Autodesk Inventor part; units mm, degrees
(part 2 of 2)
sketch "スケッチ3" plane through (0, 0, 4) normal (0, 0, 1) x (1, 0, 0)
  circle A0 centre (148.5, 105.0001) radius 6.8 projected
  arc A1 (157.8649, 90.2168) -> (159.6658, 91.5252) centre (148.5, 105.0001) ccw projected
  line L0 (159.6658, 91.5252) -> (160.4913, 90.529) projected
  arc A2 (160.4913, 90.529) -> (160.7031, 90.3266) centre (161.9356, 91.8285) ccw projected
  arc A3 (160.7031, 90.3266) -> (161.5747, 89.744) centre (164.1012, 94.4672) ccw projected
  arc A4 (161.5747, 89.744) -> (163.5573, 88.9603) centre (165.9672, 97.9557) ccw projected
  arc A5 (163.5573, 88.9603) -> (164.5398, 89.9428) centre (148.5, 105.0001) ccw projected
  arc A6 (164.5398, 89.9428) -> (163.7561, 91.9254) centre (155.5444, 87.5329) ccw projected
  arc A7 (163.7561, 91.9254) -> (163.1735, 92.797) centre (159.0329, 89.3989) ccw projected
  arc A8 (163.1735, 92.797) -> (162.9711, 93.0088) centre (161.6716, 91.5644) ccw projected
  line L1 (162.9711, 93.0088) -> (161.9749, 93.8343) projected
  arc A9 (161.9749, 93.8343) -> (163.2833, 95.6351) centre (148.5, 105.0001) ccw projected
  line L2 (163.2833, 95.6351) -> (164.3763, 94.9428) projected
  arc A10 (164.3763, 94.9428) -> (164.6402, 94.8158) centre (165.3483, 96.625) ccw projected
  arc A11 (164.6402, 94.8158) -> (165.6492, 94.531) centre (166.5924, 99.8038) ccw projected
  arc A12 (165.6492, 94.531) -> (167.7769, 94.3983) centre (167.2891, 103.6981) ccw projected
  arc A13 (167.7769, 94.3983) -> (168.4077, 95.6364) centre (148.5, 105.0001) ccw projected
  arc A14 (168.4077, 95.6364) -> (167.0497, 97.2797) centre (160.5973, 90.5647) ccw projected
  arc A15 (167.0497, 97.2797) -> (166.2263, 97.9286) centre (163.3384, 93.4173) ccw projected
  arc A16 (166.2263, 97.9286) -> (165.9684, 98.0675) centre (165.1788, 96.2923) ccw projected
  line L3 (165.9684, 98.0675) -> (164.7658, 98.5448) projected
  arc A17 (164.7658, 98.5448) -> (165.4537, 100.6618) centre (148.5, 105.0001) ccw projected
  line L4 (165.4537, 100.6618) -> (166.7071, 100.341) projected
  arc A18 (166.7071, 100.341) -> (166.9974, 100.3018) centre (167.1118, 102.2413) ccw projected
  arc A19 (166.9974, 100.3018) -> (168.045, 100.3428) centre (167.3127, 105.649) ccw projected
  arc A20 (168.045, 100.3428) -> (170.1096, 100.8741) centre (166.7718, 109.568) ccw projected
  arc A21 (170.1096, 100.8741) -> (170.327, 102.2465) centre (148.5, 105.0001) ccw projected
  arc A22 (170.327, 102.2465) -> (168.5276, 103.3897) centre (164.466, 95.0095) ccw projected
  arc A23 (168.5276, 103.3897) -> (167.5439, 103.7525) centre (166.1914, 98.5696) ccw projected
  arc A24 (167.5439, 103.7525) -> (167.2557, 103.8049) centre (167.0533, 101.8725) ccw projected
  line L5 (167.2557, 103.8049) -> (165.9645, 103.8871) projected
  arc A25 (165.9645, 103.8871) -> (165.9645, 106.1131) centre (148.5, 105.0001) ccw projected
  line L6 (165.9645, 106.1131) -> (167.2557, 106.1954) projected
  arc A26 (167.2557, 106.1954) -> (167.5439, 106.2478) centre (167.0533, 108.1277) ccw projected
  arc A27 (167.5439, 106.2478) -> (168.5276, 106.6105) centre (166.1914, 111.4307) ccw projected
  arc A28 (168.5276, 106.6105) -> (170.327, 107.7538) centre (164.466, 114.9908) ccw projected
  arc A29 (170.327, 107.7538) -> (170.1096, 109.1262) centre (148.5, 105.0001) ccw projected
  arc A30 (170.1096, 109.1262) -> (168.045, 109.6574) centre (166.7718, 100.4322) ccw projected
  arc A31 (168.045, 109.6574) -> (166.9974, 109.6984) centre (167.3127, 104.3513) ccw projected
  arc A32 (166.9974, 109.6984) -> (166.7071, 109.6592) centre (167.1118, 107.7589) ccw projected
  line L7 (166.7071, 109.6592) -> (165.4537, 109.3385) projected
  arc A33 (165.4537, 109.3385) -> (164.7658, 111.4555) centre (148.5, 105.0001) ccw projected
  line L8 (164.7658, 111.4555) -> (165.9684, 111.9328) projected
  arc A34 (165.9684, 111.9328) -> (166.2263, 112.0716) centre (165.1788, 113.708) ccw projected
  arc A35 (166.2263, 112.0716) -> (167.0497, 112.7206) centre (163.3384, 116.5829) ccw projected
  arc A36 (167.0497, 112.7206) -> (168.4077, 114.3639) centre (160.5973, 119.4356) ccw projected
  arc A37 (168.4077, 114.3639) -> (167.7769, 115.602) centre (148.5, 105.0001) ccw projected
  arc A38 (167.7769, 115.602) -> (165.6492, 115.4692) centre (167.2891, 106.3021) ccw projected
  arc A39 (165.6492, 115.4692) -> (164.6402, 115.1845) centre (166.5924, 110.1965) ccw projected
  arc A40 (164.6402, 115.1845) -> (164.3763, 115.0575) centre (165.3483, 113.3753) ccw projected
  line L9 (164.3763, 115.0575) -> (163.2833, 114.3651) projected
  arc A41 (163.2833, 114.3651) -> (161.9749, 116.166) centre (148.5, 105.0001) ccw projected
  line L10 (161.9749, 116.166) -> (162.9711, 116.9915) projected
  arc A42 (162.9711, 116.9915) -> (163.1735, 117.2033) centre (161.6716, 118.4358) ccw projected
  arc A43 (163.1735, 117.2033) -> (163.7561, 118.0749) centre (159.0329, 120.6013) ccw projected
  arc A44 (163.7561, 118.0749) -> (164.5398, 120.0574) centre (155.5444, 122.4673) ccw projected
  arc A45 (164.5398, 120.0574) -> (163.5573, 121.04) centre (148.5, 105.0001) ccw projected
  arc A46 (163.5573, 121.04) -> (161.5747, 120.2563) centre (165.9672, 112.0445) ccw projected
  arc A47 (161.5747, 120.2563) -> (160.7031, 119.6736) centre (164.1012, 115.533) ccw projected
  arc A48 (160.7031, 119.6736) -> (160.4913, 119.4713) centre (161.9356, 118.1718) ccw projected
  line L11 (160.4913, 119.4713) -> (159.6658, 118.4751) projected
  arc A49 (159.6658, 118.4751) -> (157.8649, 119.7835) centre (148.5, 105.0001) ccw projected
  line L12 (157.8649, 119.7835) -> (158.5573, 120.8764) projected
  arc A50 (158.5573, 120.8764) -> (158.6843, 121.1404) centre (156.8751, 121.8485) ccw projected
  arc A51 (158.6843, 121.1404) -> (158.9691, 122.1494) centre (153.6963, 123.0926) ccw projected
  arc A52 (158.9691, 122.1494) -> (159.1018, 124.2771) centre (149.8019, 123.7893) ccw projected
  arc A53 (159.1018, 124.2771) -> (157.8637, 124.9079) centre (148.5, 105.0001) ccw projected
  arc A54 (157.8637, 124.9079) -> (156.2204, 123.5499) centre (162.9354, 117.0974) ccw projected
  arc A55 (156.2204, 123.5499) -> (155.5715, 122.7265) centre (160.0827, 119.8386) ccw projected
  arc A56 (155.5715, 122.7265) -> (155.4326, 122.4686) centre (157.2078, 121.679) ccw projected
  line L13 (155.4326, 122.4686) -> (154.9553, 121.266) projected
  arc A57 (154.9553, 121.266) -> (152.8383, 121.9539) centre (148.5, 105.0001) ccw projected
  line L14 (152.8383, 121.9539) -> (153.159, 123.2073) projected
  arc A58 (153.159, 123.2073) -> (153.1983, 123.4975) centre (151.2588, 123.6119) ccw projected
  arc A59 (153.1983, 123.4975) -> (153.1573, 124.5452) centre (147.8511, 123.8129) ccw projected
  arc A60 (153.1573, 124.5452) -> (152.626, 126.6097) centre (143.9321, 123.272) ccw projected
  arc A61 (152.626, 126.6097) -> (151.2536, 126.8271) centre (148.5, 105.0001) ccw projected
  arc A62 (151.2536, 126.8271) -> (150.1104, 125.0278) centre (158.4906, 120.9661) ccw projected
  arc A63 (150.1104, 125.0278) -> (149.7476, 124.0441) centre (154.9305, 122.6916) ccw projected
  arc A64 (149.7476, 124.0441) -> (149.6952, 123.7559) centre (151.6276, 123.5535) ccw projected
  line L15 (149.6952, 123.7559) -> (149.613, 122.4647) projected
  arc A65 (149.613, 122.4647) -> (147.387, 122.4647) centre (148.5, 105.0001) ccw projected
  line L16 (147.387, 122.4647) -> (147.3047, 123.7559) projected
  arc A66 (147.3047, 123.7559) -> (147.2523, 124.0441) centre (145.3724, 123.5535) ccw projected
  arc A67 (147.2523, 124.0441) -> (146.8896, 125.0278) centre (142.0694, 122.6916) ccw projected
  arc A68 (146.8896, 125.0278) -> (145.7463, 126.8271) centre (138.5093, 120.9661) ccw projected
  arc A69 (145.7463, 126.8271) -> (144.3739, 126.6097) centre (148.5, 105.0001) ccw projected
  arc A70 (144.3739, 126.6097) -> (143.8427, 124.5452) centre (153.0679, 123.272) ccw projected
  arc A71 (143.8427, 124.5452) -> (143.8017, 123.4975) centre (149.1488, 123.8129) ccw projected
  arc A72 (143.8017, 123.4975) -> (143.8409, 123.2073) centre (145.7412, 123.6119) ccw projected
  line L17 (143.8409, 123.2073) -> (144.1616, 121.9539) projected
  arc A73 (144.1616, 121.9539) -> (142.0446, 121.266) centre (148.5, 105.0001) ccw projected
  line L18 (142.0446, 121.266) -> (141.5673, 122.4686) projected
  arc A74 (141.5673, 122.4686) -> (141.4285, 122.7265) centre (139.7921, 121.679) ccw projected
  arc A75 (141.4285, 122.7265) -> (140.7795, 123.5499) centre (136.9172, 119.8386) ccw projected
  arc A76 (140.7795, 123.5499) -> (139.1362, 124.9079) centre (134.0645, 117.0974) ccw projected
  arc A77 (139.1362, 124.9079) -> (137.8981, 124.2771) centre (148.5, 105.0001) ccw projected
  arc A78 (137.8981, 124.2771) -> (138.0309, 122.1494) centre (147.198, 123.7893) ccw projected
  arc A79 (138.0309, 122.1494) -> (138.3156, 121.1404) centre (143.3036, 123.0926) ccw projected
  arc A80 (138.3156, 121.1404) -> (138.4426, 120.8764) centre (140.1248, 121.8485) ccw projected
  line L19 (138.4426, 120.8764) -> (139.135, 119.7835) projected
  arc A81 (139.135, 119.7835) -> (137.3341, 118.4751) centre (148.5, 105.0001) ccw projected
  line L20 (137.3341, 118.4751) -> (136.5086, 119.4713) projected
  arc A82 (136.5086, 119.4713) -> (136.2968, 119.6736) centre (135.0643, 118.1718) ccw projected
  arc A83 (136.2968, 119.6736) -> (135.4252, 120.2563) centre (132.8988, 115.533) ccw projected
  arc A84 (135.4252, 120.2563) -> (133.4426, 121.04) centre (131.0328, 112.0445) ccw projected
  arc A85 (133.4426, 121.04) -> (132.4601, 120.0574) centre (148.5, 105.0001) ccw projected
  arc A86 (132.4601, 120.0574) -> (133.2438, 118.0749) centre (141.4555, 122.4673) ccw projected
  arc A87 (133.2438, 118.0749) -> (133.8264, 117.2033) centre (137.967, 120.6013) ccw projected
  arc A88 (133.8264, 117.2033) -> (134.0288, 116.9915) centre (135.3283, 118.4358) ccw projected
  line L21 (134.0288, 116.9915) -> (135.025, 116.166) projected
  arc A89 (135.025, 116.166) -> (133.7166, 114.3651) centre (148.5, 105.0001) ccw projected
  line L22 (133.7166, 114.3651) -> (132.6237, 115.0575) projected
  arc A90 (132.6237, 115.0575) -> (132.3597, 115.1845) centre (131.6516, 113.3753) ccw projected
  arc A91 (132.3597, 115.1845) -> (131.3507, 115.4692) centre (130.4075, 110.1965) ccw projected
  arc A92 (131.3507, 115.4692) -> (129.223, 115.602) centre (129.7108, 106.3021) ccw projected
  arc A93 (129.223, 115.602) -> (128.5922, 114.3639) centre (148.5, 105.0001) ccw projected
  arc A94 (128.5922, 114.3639) -> (129.9502, 112.7206) centre (136.4027, 119.4356) ccw projected
  arc A95 (129.9502, 112.7206) -> (130.7736, 112.0716) centre (133.6615, 116.5829) ccw projected
  arc A96 (130.7736, 112.0716) -> (131.0315, 111.9328) centre (131.8211, 113.708) ccw projected
  line L23 (131.0315, 111.9328) -> (132.2341, 111.4555) projected
  arc A97 (132.2341, 111.4555) -> (131.5462, 109.3385) centre (148.5, 105.0001) ccw projected
  line L24 (131.5462, 109.3385) -> (130.2928, 109.6592) projected
  arc A98 (130.2928, 109.6592) -> (130.0025, 109.6984) centre (129.8882, 107.7589) ccw projected
  arc A99 (130.0025, 109.6984) -> (128.9549, 109.6574) centre (129.6872, 104.3513) ccw projected
  arc A100 (128.9549, 109.6574) -> (126.8903, 109.1262) centre (130.2281, 100.4322) ccw projected
  arc A101 (126.8903, 109.1262) -> (126.673, 107.7538) centre (148.5, 105.0001) ccw projected
  arc A102 (126.673, 107.7538) -> (128.4723, 106.6105) centre (132.5339, 114.9908) ccw projected
  arc A103 (128.4723, 106.6105) -> (129.456, 106.2478) centre (130.8085, 111.4307) ccw projected
  arc A104 (129.456, 106.2478) -> (129.7442, 106.1954) centre (129.9466, 108.1277) ccw projected
  line L25 (129.7442, 106.1954) -> (131.0354, 106.1131) projected
  arc A105 (131.0354, 106.1131) -> (131.0354, 103.8871) centre (148.5, 105.0001) ccw projected
  line L26 (131.0354, 103.8871) -> (129.7442, 103.8049) projected
  arc A106 (129.7442, 103.8049) -> (129.456, 103.7525) centre (129.9466, 101.8725) ccw projected
  arc A107 (129.456, 103.7525) -> (128.4723, 103.3897) centre (130.8085, 98.5696) ccw projected
  arc A108 (128.4723, 103.3897) -> (126.673, 102.2465) centre (132.5339, 95.0095) ccw projected
  arc A109 (126.673, 102.2465) -> (126.8903, 100.8741) centre (148.5, 105.0001) ccw projected
  arc A110 (126.8903, 100.8741) -> (128.9549, 100.3428) centre (130.2281, 109.568) ccw projected
  arc A111 (128.9549, 100.3428) -> (130.0025, 100.3018) centre (129.6872, 105.649) ccw projected
  arc A112 (130.0025, 100.3018) -> (130.2928, 100.341) centre (129.8882, 102.2413) ccw projected
  line L27 (130.2928, 100.341) -> (131.5462, 100.6618) projected
  arc A113 (131.5462, 100.6618) -> (132.2341, 98.5448) centre (148.5, 105.0001) ccw projected
  line L28 (132.2341, 98.5448) -> (131.0315, 98.0675) projected
  arc A114 (131.0315, 98.0675) -> (130.7736, 97.9286) centre (131.8211, 96.2923) ccw projected
  arc A115 (130.7736, 97.9286) -> (129.9502, 97.2797) centre (133.6615, 93.4173) ccw projected
  arc A116 (129.9502, 97.2797) -> (128.5922, 95.6364) centre (136.4027, 90.5647) ccw projected
  arc A117 (128.5922, 95.6364) -> (129.223, 94.3983) centre (148.5, 105.0001) ccw projected
  arc A118 (129.223, 94.3983) -> (131.3507, 94.531) centre (129.7108, 103.6981) ccw projected
  arc A119 (131.3507, 94.531) -> (132.3597, 94.8158) centre (130.4075, 99.8038) ccw projected
  arc A120 (132.3597, 94.8158) -> (132.6237, 94.9428) centre (131.6516, 96.625) ccw projected
  line L29 (132.6237, 94.9428) -> (133.7166, 95.6351) projected
  arc A121 (133.7166, 95.6351) -> (135.025, 93.8343) centre (148.5, 105.0001) ccw projected
  line L30 (135.025, 93.8343) -> (134.0288, 93.0088) projected
  arc A122 (134.0288, 93.0088) -> (133.8264, 92.797) centre (135.3283, 91.5644) ccw projected
  arc A123 (133.8264, 92.797) -> (133.2438, 91.9254) centre (137.967, 89.3989) ccw projected
  arc A124 (133.2438, 91.9254) -> (132.4601, 89.9428) centre (141.4555, 87.5329) ccw projected
  arc A125 (132.4601, 89.9428) -> (133.4426, 88.9603) centre (148.5, 105.0001) ccw projected
  arc A126 (133.4426, 88.9603) -> (135.4252, 89.744) centre (131.0328, 97.9557) ccw projected
  arc A127 (135.4252, 89.744) -> (136.2968, 90.3266) centre (132.8988, 94.4672) ccw projected
  arc A128 (136.2968, 90.3266) -> (136.5086, 90.529) centre (135.0643, 91.8285) ccw projected
  line L31 (136.5086, 90.529) -> (137.3341, 91.5252) projected
  arc A129 (137.3341, 91.5252) -> (139.135, 90.2168) centre (148.5, 105.0001) ccw projected
  line L32 (139.135, 90.2168) -> (138.4426, 89.1238) projected
  arc A130 (138.4426, 89.1238) -> (138.3156, 88.8599) centre (140.1248, 88.1518) ccw projected
  arc A131 (138.3156, 88.8599) -> (138.0309, 87.8509) centre (143.3036, 86.9076) ccw projected
  arc A132 (138.0309, 87.8509) -> (137.8981, 85.7232) centre (147.198, 86.211) ccw projected
  arc A133 (137.8981, 85.7232) -> (139.1362, 85.0923) centre (148.5, 105.0001) ccw projected
  arc A134 (139.1362, 85.0923) -> (140.7795, 86.4504) centre (134.0645, 92.9028) ccw projected
  arc A135 (140.7795, 86.4504) -> (141.4285, 87.2738) centre (136.9172, 90.1617) ccw projected
  arc A136 (141.4285, 87.2738) -> (141.5673, 87.5317) centre (139.7921, 88.3213) ccw projected
  line L33 (141.5673, 87.5317) -> (142.0446, 88.7343) projected
  arc A137 (142.0446, 88.7343) -> (144.1616, 88.0464) centre (148.5, 105.0001) ccw projected
  line L34 (144.1616, 88.0464) -> (143.8409, 86.793) projected
  arc A138 (143.8409, 86.793) -> (143.8017, 86.5027) centre (145.7412, 86.3883) ccw projected
  arc A139 (143.8017, 86.5027) -> (143.8427, 85.4551) centre (149.1488, 86.1874) ccw projected
  arc A140 (143.8427, 85.4551) -> (144.3739, 83.3905) centre (153.0679, 86.7283) ccw projected
  arc A141 (144.3739, 83.3905) -> (145.7463, 83.1731) centre (148.5, 105.0001) ccw projected
  arc A142 (145.7463, 83.1731) -> (146.8896, 84.9725) centre (138.5093, 89.0341) ccw projected
  arc A143 (146.8896, 84.9725) -> (147.2523, 85.9562) centre (142.0694, 87.3087) ccw projected
  arc A144 (147.2523, 85.9562) -> (147.3047, 86.2444) centre (145.3724, 86.4467) ccw projected
  line L35 (147.3047, 86.2444) -> (147.387, 87.5356) projected
  arc A145 (147.387, 87.5356) -> (149.613, 87.5356) centre (148.5, 105.0001) ccw projected
  line L36 (149.613, 87.5356) -> (149.6952, 86.2444) projected
  arc A146 (149.6952, 86.2444) -> (149.7476, 85.9562) centre (151.6276, 86.4467) ccw projected
  arc A147 (149.7476, 85.9562) -> (150.1104, 84.9725) centre (154.9305, 87.3087) ccw projected
  arc A148 (150.1104, 84.9725) -> (151.2536, 83.1731) centre (158.4906, 89.0341) ccw projected
  arc A149 (151.2536, 83.1731) -> (152.626, 83.3905) centre (148.5, 105.0001) ccw projected
  arc A150 (152.626, 83.3905) -> (153.1573, 85.4551) centre (143.9321, 86.7283) ccw projected
  arc A151 (153.1573, 85.4551) -> (153.1983, 86.5027) centre (147.8511, 86.1874) ccw projected
  arc A152 (153.1983, 86.5027) -> (153.159, 86.793) centre (151.2588, 86.3883) ccw projected
  line L37 (153.159, 86.793) -> (152.8383, 88.0464) projected
  arc A153 (152.8383, 88.0464) -> (154.9553, 88.7343) centre (148.5, 105.0001) ccw projected
  line L38 (154.9553, 88.7343) -> (155.4326, 87.5317) projected
  arc A154 (155.4326, 87.5317) -> (155.5715, 87.2738) centre (157.2078, 88.3213) ccw projected
  arc A155 (155.5715, 87.2738) -> (156.2204, 86.4504) centre (160.0827, 90.1617) ccw projected
  arc A156 (156.2204, 86.4504) -> (157.8637, 85.0923) centre (162.9354, 92.9028) ccw projected
  arc A157 (157.8637, 85.0923) -> (159.1018, 85.7232) centre (148.5, 105.0001) ccw projected
  arc A158 (159.1018, 85.7232) -> (158.9691, 87.8509) centre (149.8019, 86.211) ccw projected
  arc A159 (158.9691, 87.8509) -> (158.6843, 88.8599) centre (153.6963, 86.9076) ccw projected
  arc A160 (158.6843, 88.8599) -> (158.5573, 89.1238) centre (156.8751, 88.1518) ccw projected
  line L39 (158.5573, 89.1238) -> (157.8649, 90.2168) projected
  circle A161 centre (148.5, 105.0001) radius 13.5
  circle A162 centre (148.5, 105.0001) radius 10
  circle A163 centre (148.5, 105.0001) radius 6 projected
  line L40 (147, 119.6736) -> (147, 90.1617)
  line L41 (150, 119.9822) -> (150, 90.1617)
  line L42 (132.8988, 106.5001) -> (164.1012, 106.5001)
  line L43 (133.4426, 103.5001) -> (164.5398, 103.5001)
  point P0 (0, 0)
  point P1 (138.6131, 103.5001)
  point P2 (135.0836, 103.5001)
  point P3 (147, 91.5837)
  point P4 (147, 95.1133)
  point P5 (161.9164, 103.5001)
  point P6 (158.3868, 103.5001)
  point P7 (150, 95.1133)
  point P8 (150, 91.5837)
  point P9 (158.3868, 106.5001)
  point P10 (161.9164, 106.5001)
  point P11 (150, 118.4165)
  point P12 (150, 114.887)
  point P13 (135.0836, 106.5001)
  point P14 (138.6131, 106.5001)
  point P15 (147, 114.887)
  point P16 (147, 118.4165)
  dimension "d8" = 4
  dimension "d9" = 4
  dimension "d10" = 1.5
  dimension "d11" = 3
  dimension "d12" = 1.5
  dimension "d13" = 3
  constraints: 8 end point, 2 centre point, 2 coincident, 2 vertical, 1 horizontal, 1 perpendicular
  measures "d8" radial gap between concentric circles of A65 A161
  measures "d9" radial gap between concentric circles of A162 A163
  measures "d10" distance from line of A0.centre L41
  measures "d11" distance between parallel lines of L41 L40
  measures "d12" distance from line of A9.centre L42
  measures "d13" distance between parallel lines of L42 L43
extrude "押し出し4" cut sketch "スケッチ3" against normal blind 4 contours A162 L41 A161 L42 | L43 A161 L41 A162 | A162 L42 A161 L40 | L40 A161 L43 A162
fillet "フィレット1" radius 1 16 edges at (150, 91.5837, 2) (150, 118.4165, 2) (150, 95.1133, 2) (150, 114.887, 2) (147, 95.1133, 2) (147, 114.887, 2) (147, 91.5837, 2) (147, 118.4165, 2) (138.6131, 106.5001, 2) (158.3868, 106.5001, 2) (135.0836, 106.5001, 2) (161.9164, 106.5001, 2) (138.6131, 103.5001, 2) (158.3868, 103.5001, 2) (135.0836, 103.5001, 2) (161.9164, 103.5001, 2)
sketch "スケッチ4" plane through (0, 0, 4) normal (0, 0, 1) x (1, 0, 0)
  arc A0 (151.2, 91.7729) -> (161.7272, 102.3001) centre (148.5, 105.0001) ccw projected
  arc A1 (150, 92.7527) -> (151.2, 91.7729) centre (151, 92.7527) ccw projected
  line L0 (150, 92.7527) -> (150, 94.288) projected
  arc A2 (150.7727, 95.2618) -> (150, 94.288) centre (151, 94.288) ccw projected
  arc A3 (150.7727, 95.2618) -> (158.2383, 102.7274) centre (148.5, 105.0001) ccw projected
  arc A4 (159.2121, 103.5001) -> (158.2383, 102.7274) centre (159.2121, 102.5001) ccw projected
  line L1 (159.2121, 103.5001) -> (160.7474, 103.5001) projected
  arc A5 (161.7272, 102.3001) -> (160.7474, 103.5001) centre (160.7474, 102.5001) ccw projected
  line L2 (160.7474, 106.5001) -> (159.2121, 106.5001) projected
  arc A6 (158.2383, 107.2729) -> (159.2121, 106.5001) centre (159.2121, 107.5001) ccw projected
  arc A7 (158.2383, 107.2729) -> (150.7727, 114.7384) centre (148.5, 105.0001) ccw projected
  arc A8 (150, 115.7123) -> (150.7727, 114.7384) centre (151, 115.7123) ccw projected
  line L3 (150, 115.7123) -> (150, 117.2476) projected
  arc A9 (151.2, 118.2274) -> (150, 117.2476) centre (151, 117.2476) ccw projected
  arc A10 (161.7272, 107.7001) -> (151.2, 118.2274) centre (148.5, 105.0001) ccw projected
  arc A11 (160.7474, 106.5001) -> (161.7272, 107.7001) centre (160.7474, 107.5001) ccw projected
  arc A12 (135.2727, 102.3001) -> (145.8, 91.7729) centre (148.5, 105.0001) ccw projected
  arc A13 (136.2525, 103.5001) -> (135.2727, 102.3001) centre (136.2525, 102.5001) ccw projected
  line L4 (136.2525, 103.5001) -> (137.7878, 103.5001) projected
  arc A14 (138.7617, 102.7274) -> (137.7878, 103.5001) centre (137.7878, 102.5001) ccw projected
  arc A15 (138.7617, 102.7274) -> (146.2272, 95.2618) centre (148.5, 105.0001) ccw projected
  arc A16 (147, 94.288) -> (146.2272, 95.2618) centre (146, 94.288) ccw projected
  line L5 (147, 94.288) -> (147, 92.7527) projected
  arc A17 (145.8, 91.7729) -> (147, 92.7527) centre (146, 92.7527) ccw projected
  arc A18 (146.2272, 114.7384) -> (138.7617, 107.2729) centre (148.5, 105.0001) ccw projected
  arc A19 (137.7878, 106.5001) -> (138.7617, 107.2729) centre (137.7878, 107.5001) ccw projected
  line L6 (137.7878, 106.5001) -> (136.2525, 106.5001) projected
  arc A20 (135.2727, 107.7001) -> (136.2525, 106.5001) centre (136.2525, 107.5001) ccw projected
  arc A21 (145.8, 118.2274) -> (135.2727, 107.7001) centre (148.5, 105.0001) ccw projected
  arc A22 (147, 117.2476) -> (145.8, 118.2274) centre (146, 117.2476) ccw projected
  line L7 (147, 117.2476) -> (147, 115.7123) projected
  arc A23 (146.2272, 114.7384) -> (147, 115.7123) centre (146, 115.7123) ccw projected
  circle A24 centre (148.5, 105.0001) radius 6.8 projected
  arc A25 (157.8649, 90.2168) -> (159.6658, 91.5252) centre (148.5, 105.0001) ccw projected
  line L8 (159.6658, 91.5252) -> (160.4913, 90.529) projected
  arc A26 (160.4913, 90.529) -> (160.7031, 90.3266) centre (161.9356, 91.8285) ccw projected
  arc A27 (160.7031, 90.3266) -> (161.5747, 89.744) centre (164.1012, 94.4672) ccw projected
  arc A28 (161.5747, 89.744) -> (163.5573, 88.9603) centre (165.9672, 97.9557) ccw projected
  arc A29 (163.5573, 88.9603) -> (164.5398, 89.9428) centre (148.5, 105.0001) ccw projected
  arc A30 (164.5398, 89.9428) -> (163.7561, 91.9254) centre (155.5444, 87.5329) ccw projected
  arc A31 (163.7561, 91.9254) -> (163.1735, 92.797) centre (159.0329, 89.3989) ccw projected
  arc A32 (163.1735, 92.797) -> (162.9711, 93.0088) centre (161.6716, 91.5644) ccw projected
  line L9 (162.9711, 93.0088) -> (161.9749, 93.8343) projected
  arc A33 (161.9749, 93.8343) -> (163.2833, 95.6351) centre (148.5, 105.0001) ccw projected
  line L10 (163.2833, 95.6351) -> (164.3763, 94.9428) projected
  arc A34 (164.3763, 94.9428) -> (164.6402, 94.8158) centre (165.3483, 96.625) ccw projected
  arc A35 (164.6402, 94.8158) -> (165.6492, 94.531) centre (166.5924, 99.8038) ccw projected
  arc A36 (165.6492, 94.531) -> (167.7769, 94.3983) centre (167.2891, 103.6981) ccw projected
  arc A37 (167.7769, 94.3983) -> (168.4077, 95.6364) centre (148.5, 105.0001) ccw projected
  arc A38 (168.4077, 95.6364) -> (167.0497, 97.2797) centre (160.5973, 90.5647) ccw projected
  arc A39 (167.0497, 97.2797) -> (166.2263, 97.9286) centre (163.3384, 93.4173) ccw projected
  arc A40 (166.2263, 97.9286) -> (165.9684, 98.0675) centre (165.1788, 96.2923) ccw projected
  line L11 (165.9684, 98.0675) -> (164.7658, 98.5448) projected
  arc A41 (164.7658, 98.5448) -> (165.4537, 100.6618) centre (148.5, 105.0001) ccw projected
  line L12 (165.4537, 100.6618) -> (166.7071, 100.341) projected
  arc A42 (166.7071, 100.341) -> (166.9974, 100.3018) centre (167.1118, 102.2413) ccw projected
  arc A43 (166.9974, 100.3018) -> (168.045, 100.3428) centre (167.3127, 105.649) ccw projected
  arc A44 (168.045, 100.3428) -> (170.1096, 100.8741) centre (166.7718, 109.568) ccw projected
  arc A45 (170.1096, 100.8741) -> (170.327, 102.2465) centre (148.5, 105.0001) ccw projected
  arc A46 (170.327, 102.2465) -> (168.5276, 103.3897) centre (164.466, 95.0095) ccw projected
  arc A47 (168.5276, 103.3897) -> (167.5439, 103.7525) centre (166.1914, 98.5696) ccw projected
  arc A48 (167.5439, 103.7525) -> (167.2557, 103.8049) centre (167.0533, 101.8725) ccw projected
  line L13 (167.2557, 103.8049) -> (165.9645, 103.8871) projected
  arc A49 (165.9645, 103.8871) -> (165.9645, 106.1131) centre (148.5, 105.0001) ccw projected
  line L14 (165.9645, 106.1131) -> (167.2557, 106.1954) projected
  arc A50 (167.2557, 106.1954) -> (167.5439, 106.2478) centre (167.0533, 108.1277) ccw projected
  arc A51 (167.5439, 106.2478) -> (168.5276, 106.6105) centre (166.1914, 111.4307) ccw projected
  arc A52 (168.5276, 106.6105) -> (170.327, 107.7538) centre (164.466, 114.9908) ccw projected
  arc A53 (170.327, 107.7538) -> (170.1096, 109.1262) centre (148.5, 105.0001) ccw projected
  arc A54 (170.1096, 109.1262) -> (168.045, 109.6574) centre (166.7718, 100.4322) ccw projected
  arc A55 (168.045, 109.6574) -> (166.9974, 109.6984) centre (167.3127, 104.3513) ccw projected
  arc A56 (166.9974, 109.6984) -> (166.7071, 109.6592) centre (167.1118, 107.7589) ccw projected
  line L15 (166.7071, 109.6592) -> (165.4537, 109.3385) projected
  arc A57 (165.4537, 109.3385) -> (164.7658, 111.4555) centre (148.5, 105.0001) ccw projected
  line L16 (164.7658, 111.4555) -> (165.9684, 111.9328) projected
  arc A58 (165.9684, 111.9328) -> (166.2263, 112.0716) centre (165.1788, 113.708) ccw projected
  arc A59 (166.2263, 112.0716) -> (167.0497, 112.7206) centre (163.3384, 116.5829) ccw projected
  arc A60 (167.0497, 112.7206) -> (168.4077, 114.3639) centre (160.5973, 119.4356) ccw projected
  arc A61 (168.4077, 114.3639) -> (167.7769, 115.602) centre (148.5, 105.0001) ccw projected
  arc A62 (167.7769, 115.602) -> (165.6492, 115.4692) centre (167.2891, 106.3021) ccw projected
  arc A63 (165.6492, 115.4692) -> (164.6402, 115.1845) centre (166.5924, 110.1965) ccw projected
  arc A64 (164.6402, 115.1845) -> (164.3763, 115.0575) centre (165.3483, 113.3753) ccw projected
  line L17 (164.3763, 115.0575) -> (163.2833, 114.3651) projected
  arc A65 (163.2833, 114.3651) -> (161.9749, 116.166) centre (148.5, 105.0001) ccw projected
  line L18 (161.9749, 116.166) -> (162.9711, 116.9915) projected
  arc A66 (162.9711, 116.9915) -> (163.1735, 117.2033) centre (161.6716, 118.4358) ccw projected
  arc A67 (163.1735, 117.2033) -> (163.7561, 118.0749) centre (159.0329, 120.6013) ccw projected
  arc A68 (163.7561, 118.0749) -> (164.5398, 120.0574) centre (155.5444, 122.4673) ccw projected
  arc A69 (164.5398, 120.0574) -> (163.5573, 121.04) centre (148.5, 105.0001) ccw projected
  arc A70 (163.5573, 121.04) -> (161.5747, 120.2563) centre (165.9672, 112.0445) ccw projected
  arc A71 (161.5747, 120.2563) -> (160.7031, 119.6736) centre (164.1012, 115.533) ccw projected
  arc A72 (160.7031, 119.6736) -> (160.4913, 119.4713) centre (161.9356, 118.1718) ccw projected
  line L19 (160.4913, 119.4713) -> (159.6658, 118.4751) projected
  arc A73 (159.6658, 118.4751) -> (157.8649, 119.7835) centre (148.5, 105.0001) ccw projected
  line L20 (157.8649, 119.7835) -> (158.5573, 120.8764) projected
  arc A74 (158.5573, 120.8764) -> (158.6843, 121.1404) centre (156.8751, 121.8485) ccw projected
  arc A75 (158.6843, 121.1404) -> (158.9691, 122.1494) centre (153.6963, 123.0926) ccw projected
  arc A76 (158.9691, 122.1494) -> (159.1018, 124.2771) centre (149.8019, 123.7893) ccw projected
  arc A77 (159.1018, 124.2771) -> (157.8637, 124.9079) centre (148.5, 105.0001) ccw projected
  arc A78 (157.8637, 124.9079) -> (156.2204, 123.5499) centre (162.9354, 117.0974) ccw projected
  arc A79 (156.2204, 123.5499) -> (155.5715, 122.7265) centre (160.0827, 119.8386) ccw projected
  arc A80 (155.5715, 122.7265) -> (155.4326, 122.4686) centre (157.2078, 121.679) ccw projected
  line L21 (155.4326, 122.4686) -> (154.9553, 121.266) projected
  arc A81 (154.9553, 121.266) -> (152.8383, 121.9539) centre (148.5, 105.0001) ccw projected
  line L22 (152.8383, 121.9539) -> (153.159, 123.2073) projected
  arc A82 (153.159, 123.2073) -> (153.1983, 123.4975) centre (151.2588, 123.6119) ccw projected
  arc A83 (153.1983, 123.4975) -> (153.1573, 124.5452) centre (147.8511, 123.8129) ccw projected
  arc A84 (153.1573, 124.5452) -> (152.626, 126.6097) centre (143.9321, 123.272) ccw projected
  arc A85 (152.626, 126.6097) -> (151.2536, 126.8271) centre (148.5, 105.0001) ccw projected
  arc A86 (151.2536, 126.8271) -> (150.1104, 125.0278) centre (158.4906, 120.9661) ccw projected
  arc A87 (150.1104, 125.0278) -> (149.7476, 124.0441) centre (154.9305, 122.6916) ccw projected
  arc A88 (149.7476, 124.0441) -> (149.6952, 123.7559) centre (151.6276, 123.5535) ccw projected
  line L23 (149.6952, 123.7559) -> (149.613, 122.4647) projected
  arc A89 (149.613, 122.4647) -> (147.387, 122.4647) centre (148.5, 105.0001) ccw projected
  line L24 (147.387, 122.4647) -> (147.3047, 123.7559) projected
  arc A90 (147.3047, 123.7559) -> (147.2523, 124.0441) centre (145.3724, 123.5535) ccw projected
  arc A91 (147.2523, 124.0441) -> (146.8896, 125.0278) centre (142.0694, 122.6916) ccw projected
  arc A92 (146.8896, 125.0278) -> (145.7463, 126.8271) centre (138.5093, 120.9661) ccw projected
  arc A93 (145.7463, 126.8271) -> (144.3739, 126.6097) centre (148.5, 105.0001) ccw projected
  arc A94 (144.3739, 126.6097) -> (143.8427, 124.5452) centre (153.0679, 123.272) ccw projected
  arc A95 (143.8427, 124.5452) -> (143.8017, 123.4975) centre (149.1488, 123.8129) ccw projected
  arc A96 (143.8017, 123.4975) -> (143.8409, 123.2073) centre (145.7412, 123.6119) ccw projected
  line L25 (143.8409, 123.2073) -> (144.1616, 121.9539) projected
  arc A97 (144.1616, 121.9539) -> (142.0446, 121.266) centre (148.5, 105.0001) ccw projected
  line L26 (142.0446, 121.266) -> (141.5673, 122.4686) projected
  arc A98 (141.5673, 122.4686) -> (141.4285, 122.7265) centre (139.7921, 121.679) ccw projected
  arc A99 (141.4285, 122.7265) -> (140.7795, 123.5499) centre (136.9172, 119.8386) ccw projected
  arc A100 (140.7795, 123.5499) -> (139.1362, 124.9079) centre (134.0645, 117.0974) ccw projected
  arc A101 (139.1362, 124.9079) -> (137.8981, 124.2771) centre (148.5, 105.0001) ccw projected
  arc A102 (137.8981, 124.2771) -> (138.0309, 122.1494) centre (147.198, 123.7893) ccw projected
  arc A103 (138.0309, 122.1494) -> (138.3156, 121.1404) centre (143.3036, 123.0926) ccw projected
  arc A104 (138.3156, 121.1404) -> (138.4426, 120.8764) centre (140.1248, 121.8485) ccw projected
  line L27 (138.4426, 120.8764) -> (139.135, 119.7835) projected
  arc A105 (139.135, 119.7835) -> (137.3341, 118.4751) centre (148.5, 105.0001) ccw projected
  line L28 (137.3341, 118.4751) -> (136.5086, 119.4713) projected
  arc A106 (136.5086, 119.4713) -> (136.2968, 119.6736) centre (135.0643, 118.1718) ccw projected
  arc A107 (136.2968, 119.6736) -> (135.4252, 120.2563) centre (132.8988, 115.533) ccw projected
  arc A108 (135.4252, 120.2563) -> (133.4426, 121.04) centre (131.0328, 112.0445) ccw projected
  arc A109 (133.4426, 121.04) -> (132.4601, 120.0574) centre (148.5, 105.0001) ccw projected
  arc A110 (132.4601, 120.0574) -> (133.2438, 118.0749) centre (141.4555, 122.4673) ccw projected
  arc A111 (133.2438, 118.0749) -> (133.8264, 117.2033) centre (137.967, 120.6013) ccw projected
  arc A112 (133.8264, 117.2033) -> (134.0288, 116.9915) centre (135.3283, 118.4358) ccw projected
  line L29 (134.0288, 116.9915) -> (135.025, 116.166) projected
  arc A113 (135.025, 116.166) -> (133.7166, 114.3651) centre (148.5, 105.0001) ccw projected
  line L30 (133.7166, 114.3651) -> (132.6237, 115.0575) projected
  arc A114 (132.6237, 115.0575) -> (132.3597, 115.1845) centre (131.6516, 113.3753) ccw projected
  arc A115 (132.3597, 115.1845) -> (131.3507, 115.4692) centre (130.4075, 110.1965) ccw projected
  arc A116 (131.3507, 115.4692) -> (129.223, 115.602) centre (129.7108, 106.3021) ccw projected
  arc A117 (129.223, 115.602) -> (128.5922, 114.3639) centre (148.5, 105.0001) ccw projected
  arc A118 (128.5922, 114.3639) -> (129.9502, 112.7206) centre (136.4027, 119.4356) ccw projected
  arc A119 (129.9502, 112.7206) -> (130.7736, 112.0716) centre (133.6615, 116.5829) ccw projected
  arc A120 (130.7736, 112.0716) -> (131.0315, 111.9328) centre (131.8211, 113.708) ccw projected
  line L31 (131.0315, 111.9328) -> (132.2341, 111.4555) projected
  arc A121 (132.2341, 111.4555) -> (131.5462, 109.3385) centre (148.5, 105.0001) ccw projected
  line L32 (131.5462, 109.3385) -> (130.2928, 109.6592) projected
  arc A122 (130.2928, 109.6592) -> (130.0025, 109.6984) centre (129.8882, 107.7589) ccw projected
  arc A123 (130.0025, 109.6984) -> (128.9549, 109.6574) centre (129.6872, 104.3513) ccw projected
  arc A124 (128.9549, 109.6574) -> (126.8903, 109.1262) centre (130.2281, 100.4322) ccw projected
  arc A125 (126.8903, 109.1262) -> (126.673, 107.7538) centre (148.5, 105.0001) ccw projected
  arc A126 (126.673, 107.7538) -> (128.4723, 106.6105) centre (132.5339, 114.9908) ccw projected
  arc A127 (128.4723, 106.6105) -> (129.456, 106.2478) centre (130.8085, 111.4307) ccw projected
  arc A128 (129.456, 106.2478) -> (129.7442, 106.1954) centre (129.9466, 108.1277) ccw projected
  line L33 (129.7442, 106.1954) -> (131.0354, 106.1131) projected
  arc A129 (131.0354, 106.1131) -> (131.0354, 103.8871) centre (148.5, 105.0001) ccw projected
  line L34 (131.0354, 103.8871) -> (129.7442, 103.8049) projected
  arc A130 (129.7442, 103.8049) -> (129.456, 103.7525) centre (129.9466, 101.8725) ccw projected
  arc A131 (129.456, 103.7525) -> (128.4723, 103.3897) centre (130.8085, 98.5696) ccw projected
  arc A132 (128.4723, 103.3897) -> (126.673, 102.2465) centre (132.5339, 95.0095) ccw projected
  arc A133 (126.673, 102.2465) -> (126.8903, 100.8741) centre (148.5, 105.0001) ccw projected
  arc A134 (126.8903, 100.8741) -> (128.9549, 100.3428) centre (130.2281, 109.568) ccw projected
  arc A135 (128.9549, 100.3428) -> (130.0025, 100.3018) centre (129.6872, 105.649) ccw projected
  arc A136 (130.0025, 100.3018) -> (130.2928, 100.341) centre (129.8882, 102.2413) ccw projected
  line L35 (130.2928, 100.341) -> (131.5462, 100.6618) projected
  arc A137 (131.5462, 100.6618) -> (132.2341, 98.5448) centre (148.5, 105.0001) ccw projected
  line L36 (132.2341, 98.5448) -> (131.0315, 98.0675) projected
  arc A138 (131.0315, 98.0675) -> (130.7736, 97.9286) centre (131.8211, 96.2923) ccw projected
  arc A139 (130.7736, 97.9286) -> (129.9502, 97.2797) centre (133.6615, 93.4173) ccw projected
  arc A140 (129.9502, 97.2797) -> (128.5922, 95.6364) centre (136.4027, 90.5647) ccw projected
  arc A141 (128.5922, 95.6364) -> (129.223, 94.3983) centre (148.5, 105.0001) ccw projected
  arc A142 (129.223, 94.3983) -> (131.3507, 94.531) centre (129.7108, 103.6981) ccw projected
  arc A143 (131.3507, 94.531) -> (132.3597, 94.8158) centre (130.4075, 99.8038) ccw projected
  arc A144 (132.3597, 94.8158) -> (132.6237, 94.9428) centre (131.6516, 96.625) ccw projected
  line L37 (132.6237, 94.9428) -> (133.7166, 95.6351) projected
  arc A145 (133.7166, 95.6351) -> (135.025, 93.8343) centre (148.5, 105.0001) ccw projected
  line L38 (135.025, 93.8343) -> (134.0288, 93.0088) projected
  arc A146 (134.0288, 93.0088) -> (133.8264, 92.797) centre (135.3283, 91.5644) ccw projected
  arc A147 (133.8264, 92.797) -> (133.2438, 91.9254) centre (137.967, 89.3989) ccw projected
  arc A148 (133.2438, 91.9254) -> (132.4601, 89.9428) centre (141.4555, 87.5329) ccw projected
  arc A149 (132.4601, 89.9428) -> (133.4426, 88.9603) centre (148.5, 105.0001) ccw projected
  arc A150 (133.4426, 88.9603) -> (135.4252, 89.744) centre (131.0328, 97.9557) ccw projected
  arc A151 (135.4252, 89.744) -> (136.2968, 90.3266) centre (132.8988, 94.4672) ccw projected
  arc A152 (136.2968, 90.3266) -> (136.5086, 90.529) centre (135.0643, 91.8285) ccw projected
  line L39 (136.5086, 90.529) -> (137.3341, 91.5252) projected
  arc A153 (137.3341, 91.5252) -> (139.135, 90.2168) centre (148.5, 105.0001) ccw projected
  line L40 (139.135, 90.2168) -> (138.4426, 89.1238) projected
  arc A154 (138.4426, 89.1238) -> (138.3156, 88.8599) centre (140.1248, 88.1518) ccw projected
  arc A155 (138.3156, 88.8599) -> (138.0309, 87.8509) centre (143.3036, 86.9076) ccw projected
  arc A156 (138.0309, 87.8509) -> (137.8981, 85.7232) centre (147.198, 86.211) ccw projected
  arc A157 (137.8981, 85.7232) -> (139.1362, 85.0923) centre (148.5, 105.0001) ccw projected
  arc A158 (139.1362, 85.0923) -> (140.7795, 86.4504) centre (134.0645, 92.9028) ccw projected
  arc A159 (140.7795, 86.4504) -> (141.4285, 87.2738) centre (136.9172, 90.1617) ccw projected
  arc A160 (141.4285, 87.2738) -> (141.5673, 87.5317) centre (139.7921, 88.3213) ccw projected
  line L41 (141.5673, 87.5317) -> (142.0446, 88.7343) projected
  arc A161 (142.0446, 88.7343) -> (144.1616, 88.0464) centre (148.5, 105.0001) ccw projected
  line L42 (144.1616, 88.0464) -> (143.8409, 86.793) projected
  arc A162 (143.8409, 86.793) -> (143.8017, 86.5027) centre (145.7412, 86.3883) ccw projected
  arc A163 (143.8017, 86.5027) -> (143.8427, 85.4551) centre (149.1488, 86.1874) ccw projected
  arc A164 (143.8427, 85.4551) -> (144.3739, 83.3905) centre (153.0679, 86.7283) ccw projected
  arc A165 (144.3739, 83.3905) -> (145.7463, 83.1731) centre (148.5, 105.0001) ccw projected
  arc A166 (145.7463, 83.1731) -> (146.8896, 84.9725) centre (138.5093, 89.0341) ccw projected
  arc A167 (146.8896, 84.9725) -> (147.2523, 85.9562) centre (142.0694, 87.3087) ccw projected
  arc A168 (147.2523, 85.9562) -> (147.3047, 86.2444) centre (145.3724, 86.4467) ccw projected
  line L43 (147.3047, 86.2444) -> (147.387, 87.5356) projected
  arc A169 (147.387, 87.5356) -> (149.613, 87.5356) centre (148.5, 105.0001) ccw projected
  line L44 (149.613, 87.5356) -> (149.6952, 86.2444) projected
  arc A170 (149.6952, 86.2444) -> (149.7476, 85.9562) centre (151.6276, 86.4467) ccw projected
  arc A171 (149.7476, 85.9562) -> (150.1104, 84.9725) centre (154.9305, 87.3087) ccw projected
  arc A172 (150.1104, 84.9725) -> (151.2536, 83.1731) centre (158.4906, 89.0341) ccw projected
  arc A173 (151.2536, 83.1731) -> (152.626, 83.3905) centre (148.5, 105.0001) ccw projected
  arc A174 (152.626, 83.3905) -> (153.1573, 85.4551) centre (143.9321, 86.7283) ccw projected
  arc A175 (153.1573, 85.4551) -> (153.1983, 86.5027) centre (147.8511, 86.1874) ccw projected
  arc A176 (153.1983, 86.5027) -> (153.159, 86.793) centre (151.2588, 86.3883) ccw projected
  line L45 (153.159, 86.793) -> (152.8383, 88.0464) projected
  arc A177 (152.8383, 88.0464) -> (154.9553, 88.7343) centre (148.5, 105.0001) ccw projected
  line L46 (154.9553, 88.7343) -> (155.4326, 87.5317) projected
  arc A178 (155.4326, 87.5317) -> (155.5715, 87.2738) centre (157.2078, 88.3213) ccw projected
  arc A179 (155.5715, 87.2738) -> (156.2204, 86.4504) centre (160.0827, 90.1617) ccw projected
  arc A180 (156.2204, 86.4504) -> (157.8637, 85.0923) centre (162.9354, 92.9028) ccw projected
  arc A181 (157.8637, 85.0923) -> (159.1018, 85.7232) centre (148.5, 105.0001) ccw projected
  arc A182 (159.1018, 85.7232) -> (158.9691, 87.8509) centre (149.8019, 86.211) ccw projected
  arc A183 (158.9691, 87.8509) -> (158.6843, 88.8599) centre (153.6963, 86.9076) ccw projected
  arc A184 (158.6843, 88.8599) -> (158.5573, 89.1238) centre (156.8751, 88.1518) ccw projected
  line L47 (158.5573, 89.1238) -> (157.8649, 90.2168) projected
  circle A185 centre (148.5, 105.0001) radius 6 projected
  point P0 (0, 0)
equation "\"d12\" = d10"
